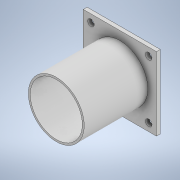
# Autodesk Inventor part: tube
Saved by Autodesk Inventor 2022.2 (Build 262287030, 287C)
## iProperties
Created: 2022-03-11
Part Number: tube
Material: Generic
Document SubType Name: Modeling
Designer: Tapendra
Density: 1 g/cm^3
Appearance: Default
Author: Tapendra
Autodesk Inventor part; units mm, degrees
ref_plane "YZ Plane" through (0, 0, 0) normal (1, 0, 0) x (0, 1, 0)
ref_plane "XZ Plane" through (0, 0, 0) normal (0, 1, 0) x (-1, 0, 0)
ref_plane "XY Plane" through (0, 0, 0) normal (0, 0, 1) x (1, 0, 0)
sketch "Sketch1" plane through (0, 0, 0) normal (0, 0, 1) x (1, 0, 0)
  line L0 (-19, 19) -> (19, 19)
  line L1 (19, 19) -> (19, -19)
  line L2 (19, -19) -> (-19, -19)
  line L3 (-19, -19) -> (-19, 19)
  line L4 (-19, 19) -> (19, -19) construction
  line L5 (19, 19) -> (-19, -19) construction
  line L6 (-11, 11) -> (11, -11) construction
  line L7 (11, 11) -> (-11, -11) construction
  circle A0 centre (0, 0) radius 13.5
  dimension "d0" = 38
  dimension "d1" = 38
  dimension "d2" = 22
  dimension "d3" = 22
  dimension "d30" = 27
  constraints: 16 end point, 4 midpoint, 2 parallel, 1 centre point, 1 coincident, 1 horizontal, 1 perpendicular
  measures "d0" distance of L0.end L1.end
  measures "d1" distance of L0.start L0.end
  measures "d2" distance of L7.start L6.end
  measures "d3" distance of L6.start L7.start
  measures "d30" diameter of A0
extrude "Extrusion1" add sketch "Sketch1" along normal mid plane 2
sketch "Sketch2" plane through (0, 0, 1) normal (0, 0, 1) x (1, 0, 0)
  line L0 (-13, 13) -> (13, -13) construction
  line L1 (13, 13) -> (-13, -13) construction
  line L2 (-11.5, -11.5) -> (11.5, 11.5) construction
  line L3 (11.5, -11.5) -> (-11.5, 11.5) construction
  circle A0 centre (0, 0) radius 13.5
  circle A1 centre (0, 0) radius 14.5
  dimension "d6" = 26
  dimension "d7" = 26
  dimension "d8" = 23
  dimension "d28" = 27
  dimension "d29" = 29
  constraints: 8 end point, 4 midpoint, 2 centre point, 2 coincident, 1 point on line
  measures "d6" distance of L1.start L0.end
  measures "d7" distance of L0.start L1.start
  measures "d8" distance of L3.start L2.end
  measures "d28" diameter of A0
  measures "d29" diameter of A1
extrude "Extrusion2" add sketch "Sketch2" along normal blind 33
sketch "Sketch3" plane through (0, 0, -1) normal (0, 0, -1) x (-1, 0, 0)
  line L0 (19, 19) -> (19, -19) projected
  line L1 (19, -19) -> (-19, -19) projected
  line L2 (-19, -19) -> (-19, 19) projected
  line L3 (-19, 19) -> (19, 19) projected
  circle A0 centre (0, 0) radius 13.5 projected
  point P0 (15, -15)
  point P1 (-15, -15)
  point P2 (15, 15)
  point P3 (-15, 15)
  dimension "d11" = 15
  dimension "d12" = 15
  dimension "d15" = 30
  dimension "d18" = 30
  constraints: 1 horizontal, 1 vertical, 3 other
  measures "d11" horizontal distance of point (15, -15) point (0, 0)
  measures "d12" horizontal distance of point (15, -15) point (0, 0)
  measures "d15" distance of point (15, -15) point (-15, -15)
  measures "d18" distance of point (15, -15) point (15, 15)
hole "Hole1" at (-15, -15, -1) at (15, -15, -1) at (-15, 15, -1) at (15, 15, -1) direction (0, 0, 1) diameter 3.4 end through all clearance for "Flat Head Machine Screw" size "M3" standard "Ansi Metric M Profile"
equation "\"d1\" = d0"
equation "\"d3\" = d2"
equation "\"d7\" = d6"
body "Solid1"
